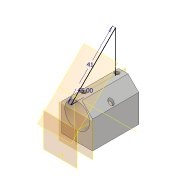
# Autodesk Inventor part: cellSTORM_v5_bluelaser_adapter
Saved by Autodesk Inventor 2019.4 (Build 234330000, 330)
## iProperties
Created: 2020-03-04
Part Number: cellSTORM_v5_bluelaser_adapter
Material: Generic
Document SubType Name: Modeling
Designer: diederichbenedict
Density: 1 g/cm^3
Appearance: Default
Author: diederichbenedict
Autodesk Inventor part; units mm, degrees
ref_plane "YZ Plane" through (0, 0, 0) normal (1, 0, 0) x (0, 1, 0)
ref_plane "XZ Plane" through (0, 0, 0) normal (0, 1, 0) x (-1, 0, 0)
ref_plane "XY Plane" through (0, 0, 0) normal (0, 0, 1) x (1, 0, 0)
ref_plane "Work Plane1" through (0, 0, 0) normal (0, 0, 1) x (1, 0, 0)
ref_plane "Work Plane2" through (0, 0, -10) normal (0, 0, 1) x (1, 0, 0)
sketch "Sketch1" plane through (0, 0, -10) normal (0, 0, 1) x (1, 0, 0)
  circle A0 centre (14.95, 17.4977) radius 7.15 projected
  line L0 (0, 2.471) -> (29.9, 2.471) projected
  line L1 (0, 2.471) -> (0, 18.471) projected
  line L2 (0, 18.471) -> (-2, 18.471) projected
  line L3 (-2, 18.471) -> (-2, -1.5) projected
  line L4 (29.9, -1.5) -> (-2, -1.5) projected
  line L5 (29.9, -1.5) -> (29.9, 2.471) projected
  line L6 (4.95, 2.471) -> (24.95, 2.471)
  line L7 (24.95, 2.471) -> (24.95, 27.471)
  line L8 (24.95, 27.471) -> (4.95, 27.471)
  line L9 (4.95, 27.471) -> (4.95, 2.471)
  circle A1 centre (14.95, 17.4977) radius 8.1
  point P0 (0, 0)
  dimension "d6" = 20
  dimension "d7" = 25
  dimension "d8" = 10
  dimension "d23" = 16.2
  constraints: 8 end point, 2 parallel, 1 centre point, 1 horizontal, 1 perpendicular, 1 point on line
  measures "d6" distance of L8.end L7.end
  measures "d7" distance of L7.end L6.end
  measures "d8" distance from line of A0.centre L9
  measures "d23" diameter of A1
extrude "Extrusion1" add sketch "Sketch1" against normal blind 30 contours L9 L8 L7 L0
sketch "Sketch2" plane through (4.95, 2.471, -10) normal (0, -1, 0) x (1, 0, 0)
  circle A0 centre (18.15, -13.73) radius 2.45 projected
  circle A1 centre (1.85, -13.73) radius 2.75 projected
  circle A2 centre (18.15, -13.73) radius 1.45
  circle A3 centre (1.85, -13.73) radius 1.45
  point P0 (-4.95, 10)
  dimension "d10" = 2.9
  dimension "d11" = 2.9
  constraints: 2 centre point, 2 coincident
  measures "d10" diameter of A2
  measures "d11" diameter of A3
extrude "Extrusion2" cut sketch "Sketch2" against normal through all contours A2 | A3
chamfer "Chamfer1" distance 7 angle 45 2 edges at (24.95, 27.471, -25) (4.95, 27.471, -25)
sketch "Sketch3" plane through (11.95, 27.471, -10) normal (0, 1, 0) x (1, 0, 0)
  line L0 (0, 0) -> (0, 30) projected
  line L1 (6, 0) -> (0, 0) projected
  line L2 (6, 30) -> (6, 0) projected
  line L3 (0, 30) -> (6, 30) projected
  circle A0 centre (2, 5.2757) radius 1.45
  circle A1 centre (2, 26.8475) radius 1.45
  point P0 (-11.95, -10)
  dimension "d17" = 2.9
  dimension "d18" = 2.9
  constraints: 2 centre point
  measures "d17" diameter of A0
  measures "d18" diameter of A1
extrude "Extrusion3" cut sketch "Sketch3" against normal blind 10 contours A0 | A1
ref_plane "Work Plane3" through (0, 27.471, -10) normal (0, -0.7071068, 0.7071068) x (1, 0, 0)
ref_plane "Work Plane4" through (11.95, 27.471, -10) normal (0, 0.7071068, 0.7071068) x (1, 0, 0)
ref_plane "Work Plane5" through (14.95, 2.471, -10) normal (1, 0, 0) x (0, 0, -1)
sketch "Sketch5" plane through (14.95, 2.471, -10) normal (1, 0, 0) x (0, 0, -1)
  line L0 (0, 23.1268) -> (30, 23.1268) projected
  line L1 (0, 6.9268) -> (30, 6.9268) projected
  line L2 (0, 23.1268) -> (-4.2183, 23.1268)
  line L3 (-4.2183, 23.1268) -> (24.7731, 52.1181)
  line L4 (24.7731, 52.1181) -> (24.7731, 23.1268)
  point P0 (-10, -2.471)
  dimension "d21" = 41
  dimension "d22" = 45
  constraints: 6 end point, 1 horizontal, 1 perpendicular, 1 point on line
  measures "d21" distance of L2.end L3.end
  measures "d22" angle of L2 L3
body "Solid1"
